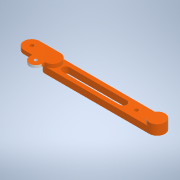
# Autodesk Inventor part: pieza4parte3
Saved by Autodesk Inventor 2021 (Build 250183000, 183)
## iProperties
Created: 2021-03-25
Part Number: pieza4parte3
Material: Genérico
Document SubType Name: Modeling
Designer: Arturo
Density: 1 g/cm^3
Appearance: Valor por defecto
Author: Arturo
Autodesk Inventor part; units mm, degrees
ref_plane "YZ Plane" through (0, 0, 0) normal (1, 0, 0) x (0, 1, 0)
ref_plane "XZ Plane" through (0, 0, 0) normal (0, 1, 0) x (-1, 0, 0)
ref_plane "XY Plane" through (0, 0, 0) normal (0, 0, 1) x (1, 0, 0)
sketch "Boceto1" plane through (0, 0, 0) normal (0, 1, 0) x (-1, 0, 0)
  arc A0 (0, 7.5) -> (0, -7.5) centre (0, 0) ccw
  circle A1 centre (20, 0) radius 1.75
  arc A2 (32.5, 3.5) -> (32.5, -3.5) centre (32.5, 0) ccw
  arc A3 (87.5, -3.5) -> (87.5, 3.5) centre (87.5, 0) ccw
  line L0 (100, 7.5) -> (0, 7.5)
  line L1 (100, -7.5) -> (0, -7.5)
  arc A4 (105, 2.5) -> (100, 7.5) centre (100, 2.5) ccw
  arc A5 (100, -7.5) -> (105, -2.5) centre (100, -2.5) ccw
  circle A6 centre (120, 0) radius 1.75
  arc A7 (120, -7.5) -> (120, 7.5) centre (120, 0) ccw
  line L2 (120, 7.5) -> (100, 7.5)
  line L3 (120, -7.5) -> (100, -7.5)
  line L4 (105, -2.5) -> (105, 2.5)
  line L5 (100, -7.5) -> (100, -10.5)
  circle A8 centre (103, -10.5) radius 1.5
  arc A9 (100, -10.5) -> (106, -10.5) centre (103, -10.5) ccw
  line L6 (106, -10.5) -> (106, -7.5)
  circle A10 centre (0, 0) radius 7.5
  line L7 (87.5, 3.5) -> (32.5, 3.5)
  line L8 (87.5, -3.5) -> (32.5, -3.5)
  point P0 (0, -7.5)
  point P1 (0, 7.5)
  point P2 (0, 7.5)
  point P3 (0, -7.5)
  dimension "d0" = 15
  dimension "d2" = 3.5
  dimension "d6" = 7
  dimension "d7" = 7
  dimension "d16" = 3.5
  dimension "d18" = 3
  dimension "d20" = 3
  dimension "d22" = 3
  dimension "d23" = 15
  dimension "d24" = 55
  dimension "d25" = 55
  constraints: 18 end point, 14 point on circle, 11 centre point, 8 tangent, 4 coincident, 1 parallel, 1 point on line
  measures "d0" diameter of A0
  measures "d2" diameter of A1
  measures "d6" diameter of A2
  measures "d7" diameter of A3
  measures "d16" diameter of A6
  measures "d18" distance of L5.end L1.start
  measures "d20" diameter of A8
  measures "d22" distance of L6.start L6.end
  measures "d23" diameter of A10
  measures "d24" distance of L7.start L7.end
  measures "d25" distance of L8.start L8.end
extrude "Extrusión1" add sketch "Boceto1" along normal blind 9.5 contours A10 A0
extrude "Extrusión2" add sketch "Boceto1" along normal blind 6 contours L0 A4 L4 A5 L1 A10
sketch "Boceto2" plane through (0, 6, 0) normal (0, 1, 0) x (1, 0, 0)
  line L0 (-100, -7.5) -> (0, -7.5) projected
  arc A0 (0, 7.5) -> (0, -7.5) centre (0, 0) ccw projected
  line L1 (0, 7.5) -> (-100, 7.5) projected
  arc A1 (-100, 7.5) -> (-105, 2.5) centre (-100, 2.5) ccw projected
  line L2 (-105, 2.5) -> (-105, -2.5) projected
  arc A2 (-105, -2.5) -> (-100, -7.5) centre (-100, -2.5) ccw projected
  circle A3 centre (-20, 0) radius 1.75 projected
  line L3 (-87.5, 3.5) -> (-32.5, 3.5) projected
  arc A4 (-32.5, -3.5) -> (-32.5, 3.5) centre (-32.5, 0) ccw projected
  line L4 (-32.5, -3.5) -> (-87.5, -3.5) projected
  arc A5 (-87.5, 3.5) -> (-87.5, -3.5) centre (-87.5, 0) ccw projected
  arc A6 (-120, 7.5) -> (-120, -7.5) centre (-120, 0) ccw
  line L5 (-120, -7.5) -> (-100, -7.5)
  line L6 (-120, 7.5) -> (-100, 7.5)
  arc A7 (-100, -7.5) -> (-100, 7.5) centre (-100, 0) ccw
  line L7 (-100, -7.5) -> (0, -7.5) projected
  line L8 (-100, -7.5) -> (-100, -10.5)
  circle A8 centre (-103, -10.5) radius 1.5
  arc A9 (-106, -10.5) -> (-100, -10.5) centre (-103, -10.5) ccw
  line L9 (-106, -10.5) -> (-106, -7.5)
  circle A10 centre (-120, 0) radius 1.75
  dimension "d31" = 15
  dimension "d32" = 20
  dimension "d33" = 20
  dimension "d35" = 3
  dimension "d39" = 3
  dimension "d40" = 3.5
  constraints: 8 end point, 6 point on circle, 5 centre point, 2 coincident, 2 tangent, 1 horizontal, 1 point on line, 1 vertical
  measures "d31" diameter of A6
  measures "d32" distance of L5.start L0.start
  measures "d33" distance of L6.start L1.end
  measures "d35" distance of L8.end L0.start
  measures "d39" distance of L9.start L9.end
  measures "d40" diameter of A10
extrude "Extrusión3" add sketch "Boceto2" along normal blind 3.5 contours L5 A6 L6 A1 L2 A2 | A2 L2 A1 A7
sketch "Boceto3" plane through (0, 9.5, 0) normal (0, 1, 0) x (1, 0, 0)
  line L0 (-105, 2.5) -> (-105, -2.5) projected
  line L1 (-120, -7.5) -> (-100, -7.5) projected
  arc A0 (-100, -7.5) -> (-100, 7.5) centre (-100, 0) ccw projected
  line L2 (-100, 7.5) -> (-120, 7.5) projected
  arc A1 (-120, 7.5) -> (-120, -7.5) centre (-120, 0) ccw projected
  circle A2 centre (-120, 0) radius 1.75 projected
  arc A3 (-100, -7.5) -> (-100, 7.5) centre (-100, 0) ccw projected
  line L3 (-100, -7.5) -> (0, -7.5) projected
  arc A4 (0, 7.5) -> (0, -7.5) centre (0, 0) ccw projected
  line L4 (0, 7.5) -> (-100, 7.5) projected
  circle A5 centre (-20, 0) radius 1.75 projected
  line L5 (-87.5, 3.5) -> (-32.5, 3.5) projected
  arc A6 (-32.5, -3.5) -> (-32.5, 3.5) centre (-32.5, 0) ccw projected
  line L6 (-32.5, -3.5) -> (-87.5, -3.5) projected
  arc A7 (-87.5, 3.5) -> (-87.5, -3.5) centre (-87.5, 0) ccw projected
  line L7 (-100, -7.5) -> (-100, -10.4769)
  line L8 (-120, -7.5) -> (-100, -7.5) projected
  line L9 (-106, -7.5) -> (-100, -7.5)
  line L10 (-111.9608, -7.5) -> (-111.9608, -10.5)
  arc A8 (-111.9608, -10.5) -> (-100, -10.4769) centre (-105.9813, -10.0037) ccw
  circle A9 centre (-105.9813, -10.0037) radius 1.5
  dimension "d52" = 3
  dimension "d53" = 6
  dimension "d54" = 3
  constraints: 6 end point, 2 centre point, 2 perpendicular, 2 point on circle, 2 point on line, 2 tangent, 1 coincident
  measures "d52" distance of L10.start L10.end
  measures "d53" radius of A8
  measures "d54" diameter of A9
extrude "Extrusión4" add sketch "Boceto3" against normal blind 2.5 contours L1 L7 A8 L10
